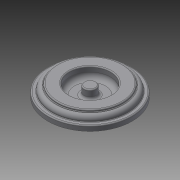
# Autodesk Inventor part: friedEggsCover
Saved by Autodesk Inventor 2014 (Build 180170000, 170)
## iProperties
Created: 2014-07-24
Part Number: friedEggsCover
Material: 一般
Document SubType Name: Modeling
Designer: hatakeyama
Density: 1 g/cm^3
Appearance: 既定
Author: hatakeyama
Autodesk Inventor part; units mm, degrees
ref_plane "YZ Plane" through (0, 0, 0) normal (1, 0, 0) x (0, 1, 0)
ref_plane "XZ Plane" through (0, 0, 0) normal (0, 1, 0) x (-1, 0, 0)
ref_plane "XY Plane" through (0, 0, 0) normal (0, 0, 1) x (1, 0, 0)
sketch "スケッチ1" plane through (0, 0, 0) normal (0, 0, 1) x (1, 0, 0)
  circle A0 centre (0, 0) radius 82
  dimension "d0" = 164
  constraints: 1 centre point, 1 coincident
  measures "d0" diameter of A0
extrude "押し出し1" add sketch "スケッチ1" along normal blind 10
sketch "スケッチ2" plane through (0, 0, 10) normal (0, 0, 1) x (1, 0, 0)
  circle A0 centre (0, 0) radius 82 projected
  circle A1 centre (0, 0) radius 74
  dimension "d3" = 8
  constraints: 1 centre point, 1 coincident
  measures "d3" radial gap between concentric circles of A1 A0
extrude "押し出し2" add sketch "スケッチ2" along normal blind 10 contours A1
sketch "スケッチ3" plane through (0, 0, 20) normal (0, 0, 1) x (1, 0, 0)
  circle A0 centre (0, 0) radius 74 projected
  circle A1 centre (0, 0) radius 64
  dimension "d6" = 128
  constraints: 1 centre point, 1 coincident
  measures "d6" diameter of A1
extrude "押し出し3" add sketch "スケッチ3" along normal blind 4 contours A1
sketch "スケッチ4" plane through (0, 0, 24) normal (0, 0, 1) x (1, 0, 0)
  circle A0 centre (0, 0) radius 64 projected
  circle A1 centre (0, 0) radius 40
  dimension "d9" = 80
  constraints: 1 centre point, 1 coincident
  measures "d9" diameter of A1
extrude "押し出し4" cut sketch "スケッチ4" against normal blind 20 contours A1
sketch "スケッチ5" plane through (0, 0, 4) normal (0, 0, 1) x (1, 0, 0)
  circle A0 centre (0, 0) radius 40 projected
  circle A1 centre (0, 0) radius 12
  dimension "d12" = 24
  constraints: 1 centre point, 1 coincident
  measures "d12" diameter of A1
extrude "押し出し5" add sketch "スケッチ5" along normal blind 17 contours A1
fillet "フィレット1" radius 2 1 edges at (-82, 0, 10)
fillet "フィレット2" radius 1 1 edges at (-74, 0, 10)
fillet "フィレット3" radius 8 1 edges at (-74, 0, 20)
fillet "フィレット4" radius 1 1 edges at (-64, 0, 20)
fillet "フィレット5" radius 2 1 edges at (-64, 0, 24)
fillet "フィレット6" radius 2 1 edges at (-40, 0, 24)
fillet "フィレット7" radius 2 1 edges at (-12, 0, 21)
fillet "フィレット8" radius 5 1 edges at (-12, 0, 4)
fillet "フィレット9" radius 10 1 edges at (-40, 0, 4)
shell "シェル1" thickness 1.5 removed faces 1 at (5.2842, -24.741, 0)
